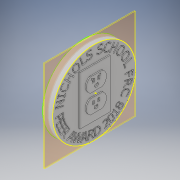
# Autodesk Inventor part: Coin Award
Saved by Autodesk Inventor 2018.2 (Build 222227000, 227)
## iProperties
Created: 2017-10-20
Part Number: Coin Award
Material: Generic
Document SubType Name: Modeling
Designer: battin.michael
Density: 1 g/cm^3
Appearance: Default
Author: battin.michael
Autodesk Inventor part; units mm, degrees
(part 1 of 3)
ref_plane "YZ Plane" through (0, 0, 0) normal (1, 0, 0) x (0, 1, 0)
ref_plane "XZ Plane" through (0, 0, 0) normal (0, 1, 0) x (-1, 0, 0)
ref_plane "XY Plane" through (0, 0, 0) normal (0, 0, 1) x (1, 0, 0)
sketch "Sketch1" plane through (0, 0, 0) normal (1, 0, 0) x (0, 1, 0)
  circle A0 centre (0, 0) radius 104.7779
  constraints: 1 centre point, 1 coincident
extrude "Extrusion1" add sketch "Sketch1" along normal blind 25.4
sketch "Sketch2" plane through (25.4, 0, 0) normal (1, 0, 0) x (0, 0, -1)
  line L0 (-38.1, 63.5) -> (38.1029, 63.5)
  line L1 (38.1029, 63.5) -> (38.1029, -60.325)
  line L2 (38.1029, -60.325) -> (-38.1, -60.325)
  line L3 (-38.1, -60.325) -> (-38.1, 63.5)
  circle A0 centre (0, 0) radius 104.7779 projected
  dimension "d56" = 66.6779
  dimension "d57" = 66.675
  constraints: 8 end point, 2 parallel, 1 horizontal, 1 perpendicular
  measures "d56" distance edge to line of A0 L3
  measures "d57" distance edge to line of A0 L1
extrude "Extrusion2" add sketch "Sketch2" along normal blind 2.54 contours L0 L1 L2 L3
sketch "Sketch3" plane through (27.94, 0, 0) normal (1, 0, 0) x (0, 0, -1)
  line L0 (-14.4399, 43.18) -> (16.0401, 43.18)
  line L1 (16.0528, 7.62) -> (-14.4272, 7.62)
  arc A0 (-14.4399, 43.18) -> (-14.4272, 7.62) centre (-4.1683, 25.4037) ccw
  arc A1 (16.0528, 7.62) -> (16.0401, 43.18) centre (5.7812, 25.3963) ccw
  line L2 (-16.0372, -4.445) -> (14.4428, -4.445) construction
  line L3 (-16.0372, -40.005) -> (14.4428, -40.005)
  arc A2 (14.4428, -40.005) -> (14.4428, -4.445) centre (4.1776, -22.225) ccw
  arc A3 (-16.0372, -4.445) -> (-16.0372, -40.005) centre (-5.7719, -22.225) ccw
  line L4 (38.1029, 63.5) -> (-38.1, 63.5) projected
  line L5 (-38.1, 63.5) -> (-38.1, -60.325) projected
  line L6 (38.1029, -60.325) -> (38.1029, 63.5) projected
  line L7 (-38.1, -60.325) -> (38.1029, -60.325) projected
  line L8 (38.1029, 63.5) -> (-38.1, 63.5) projected
  line L9 (-38.1, 63.5) -> (-38.1, -60.325) projected
  line L10 (-38.1, -60.325) -> (38.1029, -60.325) projected
  line L11 (38.1029, -60.325) -> (38.1029, 63.5) projected
  line L12 (-16.0372, -4.445) -> (14.4428, -4.445)
  line L13 (14.4428, -40.005) -> (-16.0372, -40.005)
  arc A4 (-16.0372, -4.445) -> (-16.0372, -40.005) centre (-5.7719, -22.225) ccw
  arc A5 (14.4428, -40.005) -> (14.4428, -4.445) centre (4.1776, -22.225) ccw
  point P0 (0, 0)
  dimension "d6" = 30.48
  dimension "d7" = 30.48
  dimension "d8" = 20.32
  dimension "d9" = 23.6601
  dimension "d10" = 23.6728
  dimension "d11" = 35.56
  dimension "d12" = 120
  dimension "d13" = 120
  dimension "d14" = 22.0629
  dimension "d15" = 30.48
  dimension "d16" = 30.48
  dimension "d17" = 23.6601
  dimension "d18" = 35.56
  dimension "d21" = 120
  dimension "d22" = 120
  dimension "d23" = 23.6601
  dimension "d24" = 38.1
  constraints: 12 end point, 12 point on circle, 6 centre point, 3 equal length, 3 horizontal, 1 concentric
  measures "d6" distance of L0.start L0.end
  measures "d7" distance of L1.start L1.end
  measures "d8" distance between parallel lines of L4 L0
  measures "d9" distance from line of L5 L0.start
  measures "d10" distance from line of L5 L1.end
  measures "d11" distance between parallel lines of L0 L1
  measures "d14" distance from line of L6 L0.end
  measures "d15" distance of L2.start L2.end
  measures "d16" distance of L3.start L3.end
  measures "d17" distance from line of L6 L2.end
  measures "d18" distance of L3.start L2.start
  measures "d23" distance from line of L6 L3.end
  measures "d24" distance from line of L7 A3.centre
extrude "Extrusion3" add sketch "Sketch3" along normal blind 2.54 contours L0 A1 L1 A0
ref_plane "Work Plane1" through (15.24, 0, 0) normal (1, 0, 0) x (0, 0, -1)
sketch "Sketch4" plane through (27.94, 0, 0) normal (1, 0, 0) x (0, 0, -1)
  line L0 (-14.4493, -4.4578) -> (15.0773, -4.4578)
  line L1 (16.0307, -40.005) -> (-14.4493, -40.005)
  line L2 (-38.1, -60.325) -> (38.1029, -60.325) projected
  arc A0 (16.0307, -40.005) -> (15.0773, -4.4578) centre (5.3071, -22.5062) ccw
  arc A1 (-14.4493, -4.4578) -> (-14.4493, -40.005) centre (-4.1877, -22.2314) ccw
  point P0 (0, 0)
  point P1 (16.0401, 43.18)
  dimension "d26" = 35.56
  dimension "d28" = 20.32
  dimension "d32" = 30.48
  dimension "d33" = 20.5232
  dimension "d34" = 20.5232
  dimension "d35" = 120
  dimension "d36" = 35.5472
  constraints: 4 end point, 4 point on circle, 2 centre point, 1 horizontal
  measures "d26" distance of L0.end L1.start
  measures "d28" distance between parallel lines of L2 L1
  measures "d32" distance of L1.start L1.end
  measures "d33" radius of A0
  measures "d34" radius of A1
  measures "d36" distance of L1.end L0.start
extrude "Extrusion4" [suppressed]
sketch "Sketch5" plane through (30.48, 0, 0) normal (1, 0, 0) x (0, 0, -1)
  point P0 (0, 0)
sketch "Sketch6" plane through (27.94, 0, 0) normal (1, 0, 0) x (0, 0, -1)
  line L0 (-14.4272, -4.445) -> (16.0528, -4.445)
  line L1 (16.0528, -40.005) -> (-14.4272, -40.005)
  arc A0 (-14.4272, -4.445) -> (-14.4272, -40.005) centre (-4.1767, -22.225) ccw
  arc A1 (16.0528, -40.005) -> (16.0528, -4.445) centre (5.8023, -22.225) ccw
  line L2 (38.1029, 63.5) -> (-38.1, 63.5) projected
  line L3 (38.1029, -60.325) -> (38.1029, 63.5) projected
  point P0 (0, 0)
  dimension "d37" = 35.56
  dimension "d38" = 20.5232
  dimension "d39" = 20.5232
  dimension "d42" = 103.505
  dimension "d43" = 35.56
  dimension "d44" = 30.48
  dimension "d45" = 30.48
  dimension "d58" = 22.0501
  constraints: 4 end point, 4 point on circle, 2 centre point
  measures "d37" distance of L0.end L1.start
  measures "d38" radius of A0
  measures "d39" radius of A1
  measures "d42" distance between parallel lines of L2 L1
  measures "d43" distance from line of L1 L0.start
  measures "d44" distance of L0.end L0.start
  measures "d45" distance of L1.start L1.end
  measures "d58" distance from line of L3 L0.end
extrude "Extrusion5" add sketch "Sketch6" along normal blind 2.54
sketch "Sketch7" plane through (30.48, 0, 0) normal (1, 0, 0) x (0, 0, -1)
  line L0 (-9.271, -12.3825) -> (-4.699, -12.3825)
  line L1 (-4.699, -12.3825) -> (-4.699, -20.6375)
  line L2 (-4.699, -20.6375) -> (-9.271, -20.6375)
  line L3 (-9.271, -20.6375) -> (-9.271, -12.3825)
  line L4 (-38.1, 63.5) -> (-38.1, -60.325) projected
  point P0 (0, 0)
  dimension "d46" = 4.572
  dimension "d47" = 8.255
  dimension "d50" = 28.829
  constraints: 8 end point, 2 parallel, 1 horizontal, 1 perpendicular
  measures "d46" distance of L1.end L2.end
  measures "d47" distance of L0.end L1.end
  measures "d50" distance between parallel lines of L4 L3
sketch "Sketch8" plane through (30.48, 0, 0) normal (1, 0, 0) x (0, 0, -1)
  line L0 (4.7019, -12.3237) -> (9.2739, -12.3237)
  line L1 (9.2739, -12.3237) -> (9.2739, -20.5787)
  line L2 (9.2739, -20.5787) -> (4.7019, -20.5787)
  line L3 (4.7019, -20.5787) -> (4.7019, -12.3237)
  line L4 (38.1029, -60.325) -> (38.1029, 63.5) projected
  point P0 (0, 0)
  dimension "d48" = 8.255
  dimension "d49" = 4.572
  dimension "d51" = 28.829
  constraints: 8 end point, 1 horizontal, 1 parallel, 1 perpendicular
  measures "d48" distance between parallel lines of L2 L0
  measures "d49" distance of L2.end L1.end
  measures "d51" distance between parallel lines of L4 L1
extrude "Extrusion6" cut sketch "Sketch7" against normal blind 2.54
extrude "Extrusion7" cut sketch "Sketch8" against normal blind 2.54
sketch "Sketch9" plane through (30.48, 0, 0) normal (1, 0, 0) x (0, 0, -1)
  point P0 (0, 0)
sketch "Sketch10" plane through (30.48, 0, 0) normal (1, 0, 0) x (0, 0, -1)
  line L0 (-4.7625, -25.4) -> (4.7625, -25.4)
  line L1 (4.7625, -25.4) -> (4.7625, -28.575)
  line L2 (-4.7625, -28.575) -> (-4.7625, -25.4)
  arc A0 (-4.7625, -28.575) -> (4.7625, -28.575) centre (0, -28.575) ccw
  point P0 (0, 0)
  constraints: 6 end point, 2 point on circle, 2 tangent, 1 centre point, 1 horizontal, 1 parallel, 1 perpendicular
extrude "Extrusion8" cut sketch "Sketch10" against normal blind 2.54
sketch "Sketch11" plane through (27.94, 0, 0) normal (1, 0, 0) x (0, 0, -1)
  line L0 (-1.5365, 36.5125) -> (-3.175, 36.5125)
  line L1 (-3.175, 36.5125) -> (-3.175, 28.575)
  line L2 (-3.175, 28.575) -> (-1.5365, 28.575)
  line L3 (-1.5365, 28.575) -> (-1.5365, 36.5125)
  point P0 (0, 0)
  constraints: 8 end point, 2 parallel, 1 horizontal, 1 perpendicular
sketch "Sketch12" plane through (30.48, 0, 0) normal (1, 0, 0) x (0, 0, -1)
  line L0 (-9.6418, 26.9748) -> (-4.887, 26.9748)
  line L1 (-4.887, 26.9748) -> (-4.887, 35.2298)
  line L2 (-9.6418, 35.2298) -> (-9.6418, 26.9748)
  line L3 (4.89, 26.9748) -> (9.6449, 26.9748)
  line L4 (9.6449, 26.9748) -> (9.6449, 35.2298)
  line L5 (4.89, 35.2298) -> (4.89, 26.9748)
  line L6 (16.0401, 43.18) -> (-14.4399, 43.18) projected
  line L7 (-9.6418, 35.2298) -> (-4.887, 35.2298)
  line L8 (4.89, 35.2298) -> (9.6449, 35.2298)
  point P0 (0, 0)
  dimension "d67" = 4.7549
  constraints: 16 end point, 3 equal length, 3 horizontal, 2 perpendicular, 1 point on line
  measures "d67" distance between parallel lines of L1 L2
sketch "Sketch13" plane through (30.48, 0, 0) normal (1, 0, 0) x (0, 0, -1)
  line L0 (-11.1154, 39.0904) -> (-3.164, 35.1147)
  line L1 (-3.164, 35.1147) -> (-4.8678, 31.7069)
  line L2 (-4.8678, 31.7069) -> (-12.8193, 35.6826)
  line L3 (-12.8193, 35.6826) -> (-11.1154, 39.0904)
  line L4 (-12.8193, 35.6826) -> (-9.6969, 34.1215)
  point P0 (0, 0)
  dimension "d66" = 8.89
  dimension "d68" = 3.81
  constraints: 10 end point, 2 perpendicular, 1 point on line
  measures "d66" distance between parallel lines of L1 L3
  measures "d68" distance between parallel lines of L0 L2
sketch "Sketch14" plane through (30.48, 0, 0) normal (1, 0, 0) x (0, 0, -1)
  line L0 (5.0529, 31.7537) -> (12.676, 36.3276)
  line L1 (12.676, 36.3276) -> (10.7157, 39.5946)
  line L2 (10.7157, 39.5946) -> (3.0926, 35.0208)
  line L3 (3.0926, 35.0208) -> (5.0529, 31.7537)
  point P0 (0, 0)
  dimension "d69" = 8.89
  dimension "d70" = 3.81
  constraints: 8 end point, 3 perpendicular
  measures "d69" distance between parallel lines of L1 L3
  measures "d70" distance between parallel lines of L0 L2
sketch "Sketch15" plane through (30.48, 0, 0) normal (1, 0, 0) x (0, 0, -1)
  line L0 (-4.9096, 19.5798) -> (4.568, 22.7602)
  line L1 (-4.9096, 19.5798) -> (-3.3742, 16.2781)
  line L2 (4.568, 22.7602) -> (5.7109, 19.2106)
  arc A0 (-3.3742, 16.2781) -> (5.7109, 19.2106) centre (0.987, 18.3061) ccw
  point P0 (0, 0)
  dimension "d71" = 7.091
  dimension "d72" = 3.0834
  dimension "d73" = 4.7738
  dimension "d74" = 83.612
  dimension "d75" = 89.298
  constraints: 6 end point, 2 point on circle, 1 centre point, 1 tangent
  measures "d71" angle of L2 L1
  measures "d72" distance from line of A0.centre L0
  measures "d73" distance from line of A0.centre L2
  measures "d74" angle of L0 L1
  measures "d75" angle of L2 L0
sketch "Sketch16" plane through (25.4, 0, 0) normal (1, 0, 0) x (0, 0, -1)
  point P0 (0, 0)
extrude "Extrusion9" cut sketch "Sketch15" against normal blind 2.54
extrude "Extrusion10" cut sketch "Sketch13" against normal blind 2.54
extrude "Extrusion11" cut sketch "Sketch14" against normal blind 2.54
extrude "Extrusion12" cut sketch "Sketch12" against normal blind 2.54 contours L5 L8 L4 L3
sketch "Sketch17" plane through (30.48, 0, 0) normal (1, 0, 0) x (0, 0, -1)
  line L0 (-4.7099, 31.8568) -> (-4.7099, 27.0816)
  line L1 (9.6449, 26.9748) -> (4.89, 26.9748) projected
  line L2 (-4.7099, 27.0816) -> (-9.4724, 27.0816)
  line L3 (-9.4724, 27.0816) -> (-9.4724, 34.0092)
  line L4 (-4.8678, 31.7069) -> (-12.8193, 35.6826) projected
  line L5 (-9.4724, 34.0092) -> (-4.8678, 31.7069)
  line L6 (-4.7099, 31.8568) -> (-4.7099, 32.077)
  line L7 (-4.7099, 32.077) -> (-9.4724, 34.4582)
  line L8 (-9.4724, 34.4582) -> (-9.4724, 34.0092)
  point P0 (0, 0)
  constraints: 14 end point, 3 perpendicular, 2 parallel, 1 collinear, 1 vertical
sketch "Sketch18" plane through (30.48, 0, 0) normal (1, 0, 0) x (0, 0, -1)
  point P0 (0, 0)
extrude "Extrusion13" cut sketch "Sketch17" against normal blind 2.54
ref_plane "Work Plane2" through (12.7, 0, 0) normal (1, 0, 0) x (0, 0, -1)
sketch "Sketch19" plane through (25.4, 0, 0) normal (1, 0, 0) x (0, 0, -1)
  point P0 (0, 0)
sketch "Sketch20" plane through (25.4, 0, 0) normal (1, 0, 0) x (0, 0, -1)
  circle A0 centre (0, 0) radius 88.0088
  spline S0 degree 2 poles (-64.3921, -66.344) (-64.9936, -66.9063) (-66.4769, -67.4897) (-67.2113, -67.4576) knots 0 0 0 1 2 2 2
  spline S1 degree 2 poles (-67.2113, -67.4576) (-68.1347, -67.4192) (-69.8392, -66.5753) (-70.7669, -65.5828) knots 0 0 0 1 2 2 2
  line L0 (-70.7669, -65.5828) -> (-71.7438, -64.5377)
  line L1 (-71.7438, -64.5377) -> (-75.2023, -67.7705)
  line L2 (-75.2023, -67.7705) -> (-76.3549, -66.5374)
  line L3 (-76.3549, -66.5374) -> (-67.0769, -57.8651)
  line L4 (-67.0769, -57.8651) -> (-64.8982, -60.1959)
  spline S2 degree 2 poles (-64.8982, -60.1959) (-64.1252, -61.023) (-63.3136, -62.4339) (-63.2072, -63.1656) knots 0 0 0 1 2 2 2
  spline S3 degree 2 poles (-63.2072, -63.1656) (-63.0757, -64.0147) (-63.6177, -65.6202) (-64.3921, -66.344) knots 0 0 0 1 2 2 2
  spline S4 degree 2 poles (-65.6315, -65.0935) (-65.1503, -64.6437) (-64.7528, -63.6523) (-64.8434, -63.1031) knots 0 0 0 1 2 2 2
  spline S5 degree 2 poles (-64.8434, -63.1031) (-64.922, -62.6272) (-65.495, -61.6976) (-66.0362, -61.1187) knots 0 0 0 1 2 2 2
  line L5 (-66.0362, -61.1187) -> (-66.992, -60.0962)
  line L6 (-66.992, -60.0962) -> (-70.6911, -63.5538)
  line L7 (-70.6911, -63.5538) -> (-69.904, -64.3959)
  spline S6 degree 2 poles (-69.904, -64.3959) (-69.2013, -65.1478) (-68.0962, -65.8477) (-67.4993, -65.8533) knots 0 0 0 1 2 2 2
  spline S7 degree 2 poles (-67.4993, -65.8533) (-66.9611, -65.8714) (-66.0751, -65.5081) (-65.6315, -65.0935) knots 0 0 0 1 2 2 2
  line L8 (-69.6937, -73.4893) -> (-61.2888, -63.9684)
  line L9 (-61.2888, -63.9684) -> (-55.3324, -69.2265)
  line L10 (-55.3324, -69.2265) -> (-56.3269, -70.353)
  line L11 (-56.3269, -70.353) -> (-61.0179, -66.2118)
  line L12 (-61.0179, -66.2118) -> (-63.32, -68.8197)
  line L13 (-63.32, -68.8197) -> (-58.9454, -72.6816)
  line L14 (-58.9454, -72.6816) -> (-59.9398, -73.808)
  line L15 (-59.9398, -73.808) -> (-64.3145, -69.9461)
  line L16 (-64.3145, -69.9461) -> (-67.4339, -73.4798)
  line L17 (-67.4339, -73.4798) -> (-62.7429, -77.621)
  line L18 (-62.7429, -77.621) -> (-63.7373, -78.7474)
  line L19 (-63.7373, -78.7474) -> (-69.6937, -73.4893)
  line L20 (-62.2708, -79.8763) -> (-54.8247, -69.5882)
  line L21 (-54.8247, -69.5882) -> (-48.3884, -74.2466)
  line L22 (-48.3884, -74.2466) -> (-49.2694, -75.4638)
  line L23 (-49.2694, -75.4638) -> (-54.3384, -71.795)
  line L24 (-54.3384, -71.795) -> (-56.3779, -74.613)
  line L25 (-56.3779, -74.613) -> (-51.6507, -78.0344)
  line L26 (-51.6507, -78.0344) -> (-52.5317, -79.2516)
  line L27 (-52.5317, -79.2516) -> (-57.2589, -75.8302)
  line L28 (-57.2589, -75.8302) -> (-60.0226, -79.6487)
  line L29 (-60.0226, -79.6487) -> (-54.9535, -83.3174)
  line L30 (-54.9535, -83.3174) -> (-55.8345, -84.5347)
  line L31 (-55.8345, -84.5347) -> (-62.2708, -79.8763)
  line L32 (-45.7704, -90.4564) -> (-47.6677, -89.3583)
  line L33 (-47.6677, -89.3583) -> (-48.6104, -82.9742)
  line L34 (-48.6104, -82.9742) -> (-50.285, -82.005)
  line L35 (-50.285, -82.005) -> (-52.8162, -86.3786)
  line L36 (-52.8162, -86.3786) -> (-54.277, -85.5331)
  line L37 (-54.277, -85.5331) -> (-47.9154, -74.5413)
  line L38 (-47.9154, -74.5413) -> (-45.0829, -76.1807)
  spline S8 degree 2 poles (-45.0829, -76.1807) (-44.1387, -76.7271) (-42.9835, -77.6692) (-42.621, -78.3784) knots 0 0 0 1 2 2 2
  spline S9 degree 2 poles (-42.621, -78.3784) (-42.2585, -79.0876) (-42.2658, -80.6411) (-42.7659, -81.5051) knots 0 0 0 1 2 2 2
  spline S10 degree 2 poles (-42.7659, -81.5051) (-43.4618, -82.7077) (-45.6345, -83.6263) (-46.9124, -83.4099) knots 0 0 0 1 2 2 2
  line L39 (-46.9124, -83.4099) -> (-45.7704, -90.4564)
  spline S11 degree 2 poles (-44.3561, -80.7394) (-44.0777, -80.2584) (-43.9883, -79.3232) (-44.2054, -78.8765) knots 0 0 0 1 2 2 2
  spline S12 degree 2 poles (-44.2054, -78.8765) (-44.3986, -78.4912) (-45.129, -77.8425) (-45.7347, -77.4919) knots 0 0 0 1 2 2 2
  line L40 (-45.7347, -77.4919) -> (-47.1867, -76.6516)
  line L41 (-47.1867, -76.6516) -> (-49.5787, -80.7847)
  line L42 (-49.5787, -80.7847) -> (-48.296, -81.527)
  spline S13 degree 2 poles (-48.296, -81.527) (-47.6636, -81.8931) (-46.5282, -82.2529) (-45.9797, -82.1066) knots 0 0 0 1 2 2 2
  spline S14 degree 2 poles (-45.9797, -82.1066) (-45.4838, -81.9893) (-44.686, -81.3095) (-44.3561, -80.7394) knots 0 0 0 1 2 2 2
  line L43 (-41.1552, -92.6298) -> (-32.625, -82.2927)
  line L44 (-32.625, -82.2927) -> (-30.6829, -83.0343)
  line L45 (-30.6829, -83.0343) -> (-31.2137, -96.426)
  line L46 (-31.2137, -96.426) -> (-32.8771, -95.7909)
  line L47 (-32.8771, -95.7909) -> (-32.6872, -92.0626)
  line L48 (-32.6872, -92.0626) -> (-37.2157, -90.3334)
  line L49 (-37.2157, -90.3334) -> (-39.5592, -93.2392)
  line L50 (-39.5592, -93.2392) -> (-41.1552, -92.6298)
  line L51 (-32.6059, -90.5514) -> (-32.3092, -84.2641)
  line L52 (-32.3092, -84.2641) -> (-36.2691, -89.1526)
  line L53 (-36.2691, -89.1526) -> (-32.6059, -90.5514)
  line L54 (-13.1407, -87.8693) -> (-19.1961, -99.4797)
  line L55 (-19.1961, -99.4797) -> (-21.0379, -99.0394)
  line L56 (-21.0379, -99.0394) -> (-21.1004, -88.1889)
  line L57 (-21.1004, -88.1889) -> (-25.9927, -97.8551)
  line L58 (-25.9927, -97.8551) -> (-27.8145, -97.4197)
  line L59 (-27.8145, -97.4197) -> (-28.0152, -84.3139)
  line L60 (-28.0152, -84.3139) -> (-26.3235, -84.7183)
  line L61 (-26.3235, -84.7183) -> (-26.2887, -95.5516)
  line L62 (-26.2887, -95.5516) -> (-21.3787, -85.9002)
  line L63 (-21.3787, -85.9002) -> (-19.7071, -86.2998)
  line L64 (-19.7071, -86.2998) -> (-19.7009, -97.2532)
  line L65 (-19.7009, -97.2532) -> (-14.7522, -87.4841)
  line L66 (-14.7522, -87.4841) -> (-13.1407, -87.8693)
  line L67 (-15.9288, -100.1015) -> (-10.3464, -87.9172)
  line L68 (-10.3464, -87.9172) -> (-8.2788, -88.134)
  line L69 (-8.2788, -88.134) -> (-5.3452, -101.2112)
  line L70 (-5.3452, -101.2112) -> (-7.1159, -101.0255)
  line L71 (-7.1159, -101.0255) -> (-7.892, -97.374)
  line L72 (-7.892, -97.374) -> (-12.713, -96.8685)
  line L73 (-12.713, -96.8685) -> (-14.2297, -100.2796)
  line L74 (-14.2297, -100.2796) -> (-15.9288, -100.1015)
  line L75 (-8.2024, -95.8927) -> (-9.5338, -89.7409)
  line L76 (-9.5338, -89.7409) -> (-12.1022, -95.4838)
  line L77 (-12.1022, -95.4838) -> (-8.2024, -95.8927)
  line L78 (5.8515, -101.2079) -> (3.6594, -101.2113)
  line L79 (3.6594, -101.2113) -> (-0.3621, -96.1642)
  line L80 (-0.3621, -96.1642) -> (-2.297, -96.1672)
  line L81 (-2.297, -96.1672) -> (-2.2892, -101.2204)
  line L82 (-2.2892, -101.2204) -> (-3.9771, -101.223)
  line L83 (-3.9771, -101.223) -> (-3.9965, -88.523)
  line L84 (-3.9965, -88.523) -> (-0.7238, -88.518)
  spline S15 degree 2 poles (-0.7238, -88.518) (0.3672, -88.5163) (1.8392, -88.7508) (2.5089, -89.182) knots 0 0 0 1 2 2 2
  spline S16 degree 2 poles (2.5089, -89.182) (3.1785, -89.6132) (3.9524, -90.9603) (3.954, -91.9585) knots 0 0 0 1 2 2 2
  spline S17 degree 2 poles (3.954, -91.9585) (3.9561, -93.3479) (2.5387, -95.2335) (1.325, -95.6882) knots 0 0 0 1 2 2 2
  line L85 (1.325, -95.6882) -> (5.8515, -101.2079)
  spline S18 degree 2 poles (2.1943, -92.095) (2.1934, -91.5393) (1.801, -90.6857) (1.3889, -90.4084) knots 0 0 0 1 2 2 2
  spline S19 degree 2 poles (1.3889, -90.4084) (1.0284, -90.1723) (0.0709, -89.9782) (-0.6289, -89.9793) knots 0 0 0 1 2 2 2
  line L86 (-0.6289, -89.9793) -> (-2.3065, -89.9818)
  line L87 (-2.3065, -89.9818) -> (-2.2991, -94.7572)
  line L88 (-2.2991, -94.7572) -> (-0.8171, -94.7549)
  spline S20 degree 2 poles (-0.8171, -94.7549) (-0.0864, -94.7538) (1.0761, -94.4947) (1.4769, -94.0927) knots 0 0 0 1 2 2 2
  spline S21 degree 2 poles (1.4769, -94.0927) (1.8469, -93.7422) (2.1953, -92.7537) (2.1943, -92.095) knots 0 0 0 1 2 2 2
  spline S22 degree 2 poles (16.085, -93.6581) (16.282, -95.3862) (15.198, -98.3272) (14.1106, -99.2384) knots 0 0 0 1 2 2 2
  spline S23 degree 2 poles (14.1106, -99.2384) (13.2182, -99.9512) (11.2913, -100.5851) (9.7574, -100.7599) knots 0 0 0 1 2 2 2
  line L89 (9.7574, -100.7599) -> (6.8534, -101.0909)
  line L90 (6.8534, -101.0909) -> (5.4155, -88.4725)
  line L91 (5.4155, -88.4725) -> (8.2888, -88.1451)
  spline S24 degree 2 poles (8.2888, -88.1451) (10.0681, -87.9423) (12.1533, -88.2433) (12.9227, -88.6321) knots 0 0 0 1 2 2 2
  spline S25 degree 2 poles (12.9227, -88.6321) (14.2316, -89.3013) (15.8753, -91.8175) (16.085, -93.6581) knots 0 0 0 1 2 2 2
  spline S26 degree 2 poles (14.3341, -93.8369) (14.1687, -92.3849) (12.9733, -90.4391) (11.9559, -89.9646) knots 0 0 0 1 2 2 2
  spline S27 degree 2 poles (11.9559, -89.9646) (11.2355, -89.6427) (9.6711, -89.4584) (8.5361, -89.5878) knots 0 0 0 1 2 2 2
  line L92 (8.5361, -89.5878) -> (7.2579, -89.7334)
  line L93 (7.2579, -89.7334) -> (8.3649, -99.4477)
  line L94 (8.3649, -99.4477) -> (9.6431, -99.3021)
  spline S28 degree 2 poles (9.6431, -99.3021) (10.7577, -99.1751) (12.4041, -98.6249) (13.0345, -98.0662) knots 0 0 0 1 2 2 2
  spline S29 degree 2 poles (13.0345, -98.0662) (13.8463, -97.3729) (14.5019, -95.3094) (14.3341, -93.8369) knots 0 0 0 1 2 2 2
  line L95 (31.1198, -96.3968) -> (23.5775, -98.5072)
  line L96 (23.5775, -98.5072) -> (23.0921, -96.7728)
  spline S30 degree 2 poles (23.0921, -96.7728) (23.6913, -95.7822) (24.7417, -93.9601) (25.222, -93.0028) knots 0 0 0 1 2 2 2
  spline S31 degree 2 poles (25.222, -93.0028) (26.1896, -91.0755) (26.6946, -88.9464) (26.42, -87.9652) knots 0 0 0 1 2 2 2
  spline S32 degree 2 poles (26.42, -87.9652) (26.2758, -87.4499) (25.7424, -86.7656) (25.3856, -86.5982) knots 0 0 0 1 2 2 2
  spline S33 degree 2 poles (25.3856, -86.5982) (25.0289, -86.4309) (24.2063, -86.3938) (23.7504, -86.5214) knots 0 0 0 1 2 2 2
  spline S34 degree 2 poles (23.7504, -86.5214) (23.3143, -86.6434) (22.4833, -87.1111) (22.1241, -87.3933) knots 0 0 0 1 2 2 2
  spline S35 degree 2 poles (22.1241, -87.3933) (21.816, -87.6291) (21.2828, -88.2058) (21.1234, -88.4) knots 0 0 0 1 2 2 2
  line L97 (21.1234, -88.4) -> (21.0342, -88.425)
  line L98 (21.0342, -88.425) -> (20.5461, -86.6806)
  spline S36 degree 2 poles (20.5461, -86.6806) (20.9822, -86.2914) (22.66, -85.2983) (23.4727, -85.0709) knots 0 0 0 1 2 2 2
  spline S37 degree 2 poles (23.4727, -85.0709) (25.1873, -84.5911) (27.6275, -85.864) (28.0601, -87.4101) knots 0 0 0 1 2 2 2
  spline S38 degree 2 poles (28.0601, -87.4101) (28.2626, -88.1336) (28.2639, -89.4371) (28.1108, -90.0357) knots 0 0 0 1 2 2 2
  spline S39 degree 2 poles (28.1108, -90.0357) (27.9632, -90.6541) (27.3949, -91.9459) (27.0607, -92.5845) knots 0 0 0 1 2 2 2
  spline S40 degree 2 poles (27.0607, -92.5845) (26.5233, -93.6432) (25.135, -95.9767) (24.7171, -96.6601) knots 0 0 0 1 2 2 2
  line L99 (24.7171, -96.6601) -> (30.7232, -94.9795)
  line L100 (30.7232, -94.9795) -> (31.1198, -96.3968)
  spline S41 degree 2 poles (37.8276, -87.0936) (39.0534, -90.2831) (38.3475, -93.9833) (36.4166, -94.7254) knots 0 0 0 1 2 2 2
  spline S42 degree 2 poles (36.4166, -94.7254) (34.4568, -95.4786) (31.4516, -93.1385) (30.2516, -90.0163) knots 0 0 0 1 2 2 2
  spline S43 degree 2 poles (30.2516, -90.0163) (29.0185, -86.8077) (29.7317, -83.1267) (31.6722, -82.3809) knots 0 0 0 1 2 2 2
  spline S44 degree 2 poles (31.6722, -82.3809) (33.6224, -81.6314) (36.6387, -84.0003) (37.8276, -87.0936) knots 0 0 0 1 2 2 2
  spline S45 degree 2 poles (37.1792, -91.4885) (37.1845, -90.8139) (36.6826, -88.934) (36.2137, -87.7139) knots 0 0 0 1 2 2 2
  spline S46 degree 2 poles (36.2137, -87.7139) (35.7448, -86.4939) (34.8622, -84.7713) (34.3894, -84.2583) knots 0 0 0 1 2 2 2
  spline S47 degree 2 poles (34.3894, -84.2583) (33.9167, -83.7454) (32.8409, -83.4422) (32.178, -83.697) knots 0 0 0 1 2 2 2
  spline S48 degree 2 poles (32.178, -83.697) (31.5152, -83.9517) (30.9002, -84.9048) (30.8904, -85.6252) knots 0 0 0 1 2 2 2
  spline S49 degree 2 poles (30.8904, -85.6252) (30.8828, -86.3227) (31.4188, -88.2336) (31.8655, -89.396) knots 0 0 0 1 2 2 2
  spline S50 degree 2 poles (31.8655, -89.396) (32.3455, -90.6449) (33.1416, -92.2574) (33.6425, -92.8147) knots 0 0 0 1 2 2 2
  spline S51 degree 2 poles (33.6425, -92.8147) (34.1093, -93.3409) (35.2191, -93.6751) (35.9108, -93.4093) knots 0 0 0 1 2 2 2
  spline S52 degree 2 poles (35.9108, -93.4093) (36.564, -93.1582) (37.179, -92.2052) (37.1792, -91.4885) knots 0 0 0 1 2 2 2
  line L101 (48.0313, -89.1576) -> (42.4825, -91.9138)
  line L102 (42.4825, -91.9138) -> (41.9056, -90.7524)
  line L103 (41.9056, -90.7524) -> (43.9703, -89.7268)
  line L104 (43.9703, -89.7268) -> (40.1841, -82.1041)
  line L105 (40.1841, -82.1041) -> (38.1194, -83.1297)
  line L106 (38.1194, -83.1297) -> (37.602, -82.0881)
  spline S53 degree 2 poles (37.602, -82.0881) (38.7726, -81.5067) (39.5491, -80.2936) (39.165, -79.3352) knots 0 0 0 1 2 2 2
  line L107 (39.165, -79.3352) -> (40.3448, -78.7492)
  line L108 (40.3448, -78.7492) -> (45.4359, -88.9989)
  line L109 (45.4359, -88.9989) -> (47.4545, -87.9962)
  line L110 (47.4545, -87.9962) -> (48.0313, -89.1576)
  spline S54 degree 2 poles (53.4956, -86.264) (52.6909, -86.763) (51.0719, -87.101) (50.3317, -86.9424) knots 0 0 0 1 2 2 2
  spline S55 degree 2 poles (50.3317, -86.9424) (49.6057, -86.7871) (48.3957, -85.8905) (47.9781, -85.217) knots 0 0 0 1 2 2 2
  spline S56 degree 2 poles (47.9781, -85.217) (47.4357, -84.3424) (47.4603, -82.2926) (48.0812, -81.302) knots 0 0 0 1 2 2 2
  line L111 (48.0812, -81.302) -> (48.0541, -81.2583)
  spline S57 degree 2 poles (48.0541, -81.2583) (46.9707, -81.2883) (45.5176, -80.6636) (45.0077, -79.8414) knots 0 0 0 1 2 2 2
  spline S58 degree 2 poles (45.0077, -79.8414) (44.2538, -78.6256) (45.0817, -75.8598) (46.4986, -74.9811) knots 0 0 0 1 2 2 2
  spline S59 degree 2 poles (46.4986, -74.9811) (47.968, -74.0699) (50.6982, -74.5082) (51.4467, -75.7152) knots 0 0 0 1 2 2 2
  spline S60 degree 2 poles (51.4467, -75.7152) (51.8969, -76.4411) (51.9272, -78.3842) (51.3807, -79.2801) knots 0 0 0 1 2 2 2
  line L112 (51.3807, -79.2801) -> (51.4079, -79.3238)
  spline S61 degree 2 poles (51.4079, -79.3238) (52.6237, -79.1753) (54.3756, -79.8328) (54.9939, -80.8299) knots 0 0 0 1 2 2 2
  spline S62 degree 2 poles (54.9939, -80.8299) (55.8509, -82.2118) (55, -85.3311) (53.4956, -86.264) knots 0 0 0 1 2 2 2
  spline S63 degree 2 poles (53.5938, -81.8919) (53.1816, -81.2272) (52.1686, -80.7654) (51.1757, -80.8241) knots 0 0 0 1 2 2 2
  spline S64 degree 2 poles (51.1757, -80.8241) (50.844, -80.8361) (49.8212, -81.0223) (49.1749, -81.1324) knots 0 0 0 1 2 2 2
  spline S65 degree 2 poles (49.1749, -81.1324) (48.8243, -81.8948) (48.9126, -83.4628) (49.3736, -84.2062) knots 0 0 0 1 2 2 2
  spline S66 degree 2 poles (49.3736, -84.2062) (49.9811, -85.1858) (51.9538, -85.7306) (52.8459, -85.1773) knots 0 0 0 1 2 2 2
  spline S67 degree 2 poles (52.8459, -85.1773) (53.7555, -84.6132) (54.1796, -82.8365) (53.5938, -81.8919) knots 0 0 0 1 2 2 2
  spline S68 degree 2 poles (50.0406, -76.6113) (49.5904, -75.8854) (48.0175, -75.5166) (47.1516, -76.0536) knots 0 0 0 1 2 2 2
  spline S69 degree 2 poles (47.1516, -76.0536) (46.3644, -76.5417) (45.8956, -78.0314) (46.3566, -78.7748) knots 0 0 0 1 2 2 2
  spline S70 degree 2 poles (46.3566, -78.7748) (46.6875, -79.3084) (47.6645, -79.7318) (48.365, -79.7092) knots 0 0 0 1 2 2 2
  spline S71 degree 2 poles (48.365, -79.7092) (48.6596, -79.696) (49.8525, -79.5496) (50.3045, -79.4389) knots 0 0 0 1 2 2 2
  spline S72 degree 2 poles (50.3045, -79.4389) (50.6359, -78.5673) (50.4474, -77.2673) (50.0406, -76.6113) knots 0 0 0 1 2 2 2
  line L113 (-52.1152, 71.0647) -> (-53.5825, 69.8676)
  line L114 (-53.5825, 69.8676) -> (-64.859, 74.8001)
  line L115 (-64.859, 74.8001) -> (-57.9365, 66.3153)
  line L116 (-57.9365, 66.3153) -> (-59.1566, 65.3199)
  line L117 (-59.1566, 65.3199) -> (-67.1851, 75.1603)
  line L118 (-67.1851, 75.1603) -> (-65.327, 76.6762)
  line L119 (-65.327, 76.6762) -> (-55.0073, 72.1187)
  line L120 (-55.0073, 72.1187) -> (-61.3638, 79.9097)
  line L121 (-61.3638, 79.9097) -> (-60.1437, 80.9051)
  line L122 (-60.1437, 80.9051) -> (-52.1152, 71.0647)
  line L123 (-46.2675, 74.9059) -> (-50.3792, 72.205)
  line L124 (-50.3792, 72.205) -> (-51.0911, 73.2888)
  line L125 (-51.0911, 73.2888) -> (-49.7406, 74.1759)
  line L126 (-49.7406, 74.1759) -> (-55.2893, 82.623)
  line L127 (-55.2893, 82.623) -> (-56.6398, 81.7359)
  line L128 (-56.6398, 81.7359) -> (-57.3518, 82.8197)
  line L129 (-57.3518, 82.8197) -> (-53.2401, 85.5206)
  line L130 (-53.2401, 85.5206) -> (-52.5281, 84.4368)
  line L131 (-52.5281, 84.4368) -> (-53.8786, 83.5496)
  line L132 (-53.8786, 83.5496) -> (-48.3299, 75.1026)
  line L133 (-48.3299, 75.1026) -> (-46.9794, 75.9897)
  line L134 (-46.9794, 75.9897) -> (-46.2675, 74.9059)
  spline S73 degree 2 poles (-40.0131, 78.139) (-41.1059, 77.5635) (-43.3429, 77.3277) (-44.4051, 77.7105) knots 0 0 0 1 2 2 2
  spline S74 degree 2 poles (-44.4051, 77.7105) (-45.4626, 78.0841) (-47.3511, 79.8812) (-48.0992, 81.3018) knots 0 0 0 1 2 2 2
  spline S75 degree 2 poles (-48.0992, 81.3018) (-48.8425, 82.7133) (-49.226, 85.1866) (-48.9506, 86.3202) knots 0 0 0 1 2 2 2
  spline S76 degree 2 poles (-48.9506, 86.3202) (-48.6747, 87.4309) (-47.2525, 89.1918) (-46.1142, 89.7912) knots 0 0 0 1 2 2 2
  spline S77 degree 2 poles (-46.1142, 89.7912) (-45.5496, 90.0885) (-44.4707, 90.4473) (-43.9846, 90.5404) knots 0 0 0 1 2 2 2
  spline S78 degree 2 poles (-43.9846, 90.5404) (-43.5581, 90.6138) (-42.6248, 90.6749) (-42.146, 90.6712) knots 0 0 0 1 2 2 2
  line L135 (-42.146, 90.6712) -> (-41.1965, 88.8681)
  line L136 (-41.1965, 88.8681) -> (-41.3149, 88.8058)
  spline S79 degree 2 poles (-41.3149, 88.8058) (-41.6111, 88.8824) (-42.4989, 89.0663) (-43.0746, 89.0772) knots 0 0 0 1 2 2 2
  spline S80 degree 2 poles (-43.0746, 89.0772) (-43.6272, 89.0886) (-44.7963, 88.8568) (-45.4519, 88.5115) knots 0 0 0 1 2 2 2
  spline S81 degree 2 poles (-45.4519, 88.5115) (-46.1713, 88.1327) (-47.1436, 86.8647) (-47.329, 86.0459) knots 0 0 0 1 2 2 2
  spline S82 degree 2 poles (-47.329, 86.0459) (-47.5004, 85.2229) (-47.1126, 83.2054) (-46.542, 82.1218) knots 0 0 0 1 2 2 2
  spline S83 degree 2 poles (-46.542, 82.1218) (-45.933, 80.9653) (-44.5, 79.5914) (-43.7152, 79.2718) knots 0 0 0 1 2 2 2
  spline S84 degree 2 poles (-43.7152, 79.2718) (-42.9492, 78.9657) (-41.3861, 79.0676) (-40.6758, 79.4417) knots 0 0 0 1 2 2 2
  spline S85 degree 2 poles (-40.6758, 79.4417) (-40.0293, 79.7821) (-39.0952, 80.6811) (-38.7919, 81.1432) knots 0 0 0 1 2 2 2
  spline S86 degree 2 poles (-38.7919, 81.1432) (-38.5068, 81.5958) (-38.1556, 82.4088) (-38.0737, 82.6729) knots 0 0 0 1 2 2 2
  line L137 (-38.0737, 82.6729) -> (-37.9645, 82.7305)
  line L138 (-37.9645, 82.7305) -> (-37.0246, 80.9456)
  spline S87 degree 2 poles (-37.0246, 80.9456) (-37.3068, 80.576) (-37.7946, 79.912) (-38.1823, 79.5218) knots 0 0 0 1 2 2 2
  spline S88 degree 2 poles (-38.1823, 79.5218) (-38.5878, 79.0989) (-39.3392, 78.4938) (-40.0131, 78.139) knots 0 0 0 1 2 2 2
  line L139 (-26.5432, 84.0373) -> (-28.1239, 83.4454)
  line L140 (-28.1239, 83.4454) -> (-30.3036, 89.2669)
  line L141 (-30.3036, 89.2669) -> (-35.7781, 87.217)
  line L142 (-35.7781, 87.217) -> (-33.5984, 81.3955)
  line L143 (-33.5984, 81.3955) -> (-35.179, 80.8037)
  line L144 (-35.179, 80.8037) -> (-39.6324, 92.6973)
  line L145 (-39.6324, 92.6973) -> (-38.0518, 93.2891)
  line L146 (-38.0518, 93.2891) -> (-36.305, 88.6242)
  line L147 (-36.305, 88.6242) -> (-30.8305, 90.6741)
  line L148 (-30.8305, 90.6741) -> (-32.5772, 95.339)
  line L149 (-32.5772, 95.339) -> (-30.9966, 95.9308)
  line L150 (-30.9966, 95.9308) -> (-26.5432, 84.0373)
  spline S89 degree 2 poles (-17.7919, 97.7357) (-16.9038, 97.0704) (-15.5786, 94.8368) (-15.2307, 93.2905) knots 0 0 0 1 2 2 2
  spline S90 degree 2 poles (-15.2307, 93.2905) (-14.892, 91.7844) (-15.1062, 89.1728) (-15.6439, 88.1868) knots 0 0 0 1 2 2 2
  spline S91 degree 2 poles (-15.6439, 88.1868) (-16.2128, 87.1517) (-18.0458, 85.8743) (-19.2607, 85.601) knots 0 0 0 1 2 2 2
  spline S92 degree 2 poles (-19.2607, 85.601) (-20.5158, 85.3187) (-22.716, 85.7205) (-23.6364, 86.389) knots 0 0 0 1 2 2 2
  spline S93 degree 2 poles (-23.6364, 86.389) (-24.5346, 87.052) (-25.842, 89.3001) (-26.1853, 90.8263) knots 0 0 0 1 2 2 2
  spline S94 degree 2 poles (-26.1853, 90.8263) (-26.5354, 92.3827) (-26.2953, 94.9262) (-25.7744, 95.9401) knots 0 0 0 1 2 2 2
  spline S95 degree 2 poles (-25.7744, 95.9401) (-25.2366, 96.926) (-23.4104, 98.2335) (-22.1653, 98.5136) knots 0 0 0 1 2 2 2
  spline S96 degree 2 poles (-22.1653, 98.5136) (-20.9002, 98.7981) (-18.6732, 98.3708) (-17.7919, 97.7357) knots 0 0 0 1 2 2 2
  spline S97 degree 2 poles (-16.9477, 92.9043) (-17.2233, 94.1293) (-18.1823, 95.9073) (-18.8043, 96.4214) knots 0 0 0 1 2 2 2
  spline S98 degree 2 poles (-18.8043, 96.4214) (-19.4409, 96.9533) (-20.9711, 97.2843) (-21.8346, 97.09) knots 0 0 0 1 2 2 2
  spline S99 degree 2 poles (-21.8346, 97.09) (-22.7282, 96.889) (-23.9336, 95.9638) (-24.2967, 95.1859) knots 0 0 0 1 2 2 2
  spline S100 degree 2 poles (-24.2967, 95.1859) (-24.6464, 94.4427) (-24.7394, 92.4175) (-24.4683, 91.2126) knots 0 0 0 1 2 2 2
  spline S101 degree 2 poles (-24.4683, 91.2126) (-23.9195, 88.7727) (-21.2884, 86.6429) (-19.5714, 87.0291) knots 0 0 0 1 2 2 2
  spline S102 degree 2 poles (-19.5714, 87.0291) (-17.8544, 87.4153) (-16.3989, 90.4644) (-16.9477, 92.9043) knots 0 0 0 1 2 2 2
  line L151 (-4.6682, 87.9901) -> (-11.9886, 87.242)
  line L152 (-11.9886, 87.242) -> (-13.2798, 99.8761)
  line L153 (-13.2798, 99.8761) -> (-11.6007, 100.0478)
  line L154 (-11.6007, 100.0478) -> (-10.4623, 88.9084)
  line L155 (-10.4623, 88.9084) -> (-4.8209, 89.4849)
  line L156 (-4.8209, 89.4849) -> (-4.6682, 87.9901)
  spline S103 degree 2 poles (0.1976, 87.7821) (-1.1815, 87.7858) (-3.1148, 88.3673) (-3.9679, 88.7812) knots 0 0 0 1 2 2 2
  line L157 (-3.9679, 88.7812) -> (-3.9623, 90.9013)
  line L158 (-3.9623, 90.9013) -> (-3.8388, 90.901)
  spline S104 degree 2 poles (-3.8388, 90.901) (-3.0072, 90.1166) (-0.8997, 89.2465) (0.078, 89.2439) knots 0 0 0 1 2 2 2
  spline S105 degree 2 poles (0.078, 89.2439) (1.4776, 89.2402) (2.9113, 90.3993) (2.9138, 91.3564) knots 0 0 0 1 2 2 2
  spline S106 degree 2 poles (2.9138, 91.3564) (2.9158, 92.118) (2.1671, 93.0669) (1.3547, 93.3057) knots 0 0 0 1 2 2 2
  spline S107 degree 2 poles (1.3547, 93.3057) (0.7685, 93.472) (-0.2086, 93.701) (-0.9389, 93.8882) knots 0 0 0 1 2 2 2
  spline S108 degree 2 poles (-0.9389, 93.8882) (-1.5971, 94.0649) (-2.6351, 94.5925) (-3.0354, 95.0156) knots 0 0 0 1 2 2 2
  spline S109 degree 2 poles (-3.0354, 95.0156) (-3.4253, 95.4386) (-3.8546, 96.5718) (-3.8526, 97.3128) knots 0 0 0 1 2 2 2
  spline S110 degree 2 poles (-3.8526, 97.3128) (-3.8485, 98.8566) (-1.4347, 100.9394) (0.4281, 100.9344) knots 0 0 0 1 2 2 2
  spline S111 degree 2 poles (0.4281, 100.9344) (1.4985, 100.9316) (3.391, 100.5046) (4.203, 100.101) knots 0 0 0 1 2 2 2
  line L159 (4.203, 100.101) -> (4.1976, 98.0838)
  line L160 (4.1976, 98.0838) -> (4.0741, 98.0842)
  spline S112 degree 2 poles (4.0741, 98.0842) (3.4684, 98.6415) (1.5769, 99.4699) (0.5374, 99.4727) knots 0 0 0 1 2 2 2
  spline S113 degree 2 poles (0.5374, 99.4727) (-0.6358, 99.4758) (-2.0899, 98.3785) (-2.0923, 97.4831) knots 0 0 0 1 2 2 2
  spline S114 degree 2 poles (-2.0923, 97.4831) (-2.0944, 96.6803) (-1.2427, 95.7209) (-0.4406, 95.5027) knots 0 0 0 1 2 2 2
  spline S115 degree 2 poles (-0.4406, 95.5027) (0.0942, 95.3572) (1.6473, 94.9825) (2.1615, 94.8268) knots 0 0 0 1 2 2 2
  spline S116 degree 2 poles (2.1615, 94.8268) (3.4674, 94.4219) (4.6776, 92.8029) (4.6744, 91.6193) knots 0 0 0 1 2 2 2
  spline S117 degree 2 poles (4.6744, 91.6193) (4.6724, 90.868) (4.0614, 89.4288) (3.5146, 88.926) knots 0 0 0 1 2 2 2
  spline S118 degree 2 poles (3.5146, 88.926) (2.9059, 88.3718) (1.3605, 87.779) (0.1976, 87.7821) knots 0 0 0 1 2 2 2
  spline S119 degree 2 poles (15.2495, 86.4476) (13.8914, 86.6878) (12.0865, 87.5922) (11.317, 88.1463) knots 0 0 0 1 2 2 2
  line L161 (11.317, 88.1463) -> (11.6862, 90.234)
  line L162 (11.6862, 90.234) -> (11.8078, 90.2125)
  spline S120 degree 2 poles (11.8078, 90.2125) (12.4925, 89.2972) (14.4195, 88.0785) (15.3823, 87.9083) knots 0 0 0 1 2 2 2
  spline S121 degree 2 poles (15.3823, 87.9083) (16.7606, 87.6645) (18.3718, 88.5606) (18.5385, 89.5032) knots 0 0 0 1 2 2 2
  spline S122 degree 2 poles (18.5385, 89.5032) (18.6711, 90.2531) (18.0961, 91.3163) (17.3367, 91.691) knots 0 0 0 1 2 2 2
  spline S123 degree 2 poles (17.3367, 91.691) (16.7877, 91.9553) (15.8644, 92.3485) (15.1771, 92.6581) knots 0 0 0 1 2 2 2
  spline S124 degree 2 poles (15.1771, 92.6581) (14.5589, 92.9451) (13.6267, 93.643) (13.305, 94.1284) knots 0 0 0 1 2 2 2
  spline S125 degree 2 poles (13.305, 94.1284) (12.9933, 94.612) (12.7648, 95.802) (12.8938, 96.5317) knots 0 0 0 1 2 2 2
  spline S126 degree 2 poles (12.8938, 96.5317) (13.1626, 98.0519) (15.8979, 99.6899) (17.7322, 99.3655) knots 0 0 0 1 2 2 2
  spline S127 degree 2 poles (17.7322, 99.3655) (18.7862, 99.1791) (20.5775, 98.4339) (21.3082, 97.8971) knots 0 0 0 1 2 2 2
  line L163 (21.3082, 97.8971) -> (20.957, 95.9107)
  line L164 (20.957, 95.9107) -> (20.8354, 95.9322)
  spline S128 degree 2 poles (20.8354, 95.9322) (20.3342, 96.5852) (18.6128, 97.7257) (17.5893, 97.9067) knots 0 0 0 1 2 2 2
  spline S129 degree 2 poles (17.5893, 97.9067) (16.4339, 98.111) (14.8132, 97.2793) (14.6573, 96.3976) knots 0 0 0 1 2 2 2
  spline S130 degree 2 poles (14.6573, 96.3976) (14.5175, 95.6071) (15.192, 94.5158) (15.9449, 94.1632) knots 0 0 0 1 2 2 2
  spline S131 degree 2 poles (15.9449, 94.1632) (16.4468, 93.9282) (17.9126, 93.2927) (18.3924, 93.0511) knots 0 0 0 1 2 2 2
  spline S132 degree 2 poles (18.3924, 93.0511) (19.6096, 92.4283) (20.5242, 90.6257) (20.3181, 89.4602) knots 0 0 0 1 2 2 2
  spline S133 degree 2 poles (20.3181, 89.4602) (20.1873, 88.7204) (19.3384, 87.4073) (18.7135, 87.0057) knots 0 0 0 1 2 2 2
  spline S134 degree 2 poles (18.7135, 87.0057) (18.0188, 86.5641) (16.3947, 86.2451) (15.2495, 86.4476) knots 0 0 0 1 2 2 2
  spline S135 degree 2 poles (26.0399, 83.8372) (24.8564, 84.19) (23.0924, 85.5857) (22.6007, 86.6022) knots 0 0 0 1 2 2 2
  spline S136 degree 2 poles (22.6007, 86.6022) (22.1061, 87.6088) (22.0129, 90.214) (22.4715, 91.7526) knots 0 0 0 1 2 2 2
  spline S137 degree 2 poles (22.4715, 91.7526) (22.9273, 93.2814) (24.3827, 95.3175) (25.3723, 95.9354) knots 0 0 0 1 2 2 2
  spline S138 degree 2 poles (25.3723, 95.9354) (26.3462, 96.5364) (28.5943, 96.8005) (29.8271, 96.433) knots 0 0 0 1 2 2 2
  spline S139 degree 2 poles (29.8271, 96.433) (30.4386, 96.2507) (31.4607, 95.7527) (31.8733, 95.4794) knots 0 0 0 1 2 2 2
  spline S140 degree 2 poles (31.8733, 95.4794) (32.2296, 95.2335) (32.9394, 94.6246) (33.2791, 94.287) knots 0 0 0 1 2 2 2
  line L165 (33.2791, 94.287) -> (32.6969, 92.3342)
  line L166 (32.6969, 92.3342) -> (32.5687, 92.3724)
  spline S141 degree 2 poles (32.5687, 92.3724) (32.4105, 92.6344) (31.9045, 93.3866) (31.5006, 93.797) knots 0 0 0 1 2 2 2
  spline S142 degree 2 poles (31.5006, 93.797) (31.1135, 94.1916) (30.1158, 94.8435) (29.4056, 95.0551) knots 0 0 0 1 2 2 2
  spline S143 degree 2 poles (29.4056, 95.0551) (28.6265, 95.2874) (27.0447, 95.0609) (26.3397, 94.6053) knots 0 0 0 1 2 2 2
  spline S144 degree 2 poles (26.3397, 94.6053) (25.6416, 94.1368) (24.508, 92.4235) (24.1581, 91.2498) knots 0 0 0 1 2 2 2
  spline S145 degree 2 poles (24.1581, 91.2498) (23.7847, 89.9973) (23.8482, 88.013) (24.1857, 87.2358) knots 0 0 0 1 2 2 2
  spline S146 degree 2 poles (24.1857, 87.2358) (24.5192, 86.4813) (25.7079, 85.4611) (26.4772, 85.2318) knots 0 0 0 1 2 2 2
  spline S147 degree 2 poles (26.4772, 85.2318) (27.1774, 85.023) (28.4737, 85.0125) (29.0137, 85.1307) knots 0 0 0 1 2 2 2
  spline S148 degree 2 poles (29.0137, 85.1307) (29.534, 85.2548) (30.3536, 85.5904) (30.5969, 85.722) knots 0 0 0 1 2 2 2
  line L167 (30.5969, 85.722) -> (30.7152, 85.6867)
  line L168 (30.7152, 85.6867) -> (30.1389, 83.7536)
  spline S149 degree 2 poles (30.1389, 83.7536) (29.6787, 83.6867) (28.8657, 83.5532) (28.3156, 83.5454) knots 0 0 0 1 2 2 2
  spline S150 degree 2 poles (28.3156, 83.5454) (27.7301, 83.5266) (26.7698, 83.6196) (26.0399, 83.8372) knots 0 0 0 1 2 2 2
  line L169 (39.7933, 78.6339) -> (38.2495, 79.3162)
  line L170 (38.2495, 79.3162) -> (40.7623, 85.0019)
  line L171 (40.7623, 85.0019) -> (35.4155, 87.3649)
  line L172 (35.4155, 87.3649) -> (32.9027, 81.6792)
  line L173 (32.9027, 81.6792) -> (31.3589, 82.3615)
  line L174 (31.3589, 82.3615) -> (36.4927, 93.9777)
  line L175 (36.4927, 93.9777) -> (38.0365, 93.2954)
  line L176 (38.0365, 93.2954) -> (36.0229, 88.7393)
  line L177 (36.0229, 88.7393) -> (41.3697, 86.3763)
  line L178 (41.3697, 86.3763) -> (43.3833, 90.9323)
  line L179 (43.3833, 90.9323) -> (44.9271, 90.2501)
  line L180 (44.9271, 90.2501) -> (39.7933, 78.6339)
  spline S151 degree 2 poles (55.6283, 82.3062) (55.7979, 81.2096) (55.1832, 78.6862) (54.3506, 77.3377) knots 0 0 0 1 2 2 2
  spline S152 degree 2 poles (54.3506, 77.3377) (53.5395, 76.0241) (51.5601, 74.3071) (50.4862, 73.9783) knots 0 0 0 1 2 2 2
  spline S153 degree 2 poles (50.4862, 73.9783) (49.3557, 73.6362) (47.1522, 74.0049) (46.0926, 74.6592) knots 0 0 0 1 2 2 2
  spline S154 degree 2 poles (46.0926, 74.6592) (44.9979, 75.335) (43.7062, 77.1608) (43.5157, 78.2823) knots 0 0 0 1 2 2 2
  spline S155 degree 2 poles (43.5157, 78.2823) (43.3373, 79.3843) (43.9749, 81.9056) (44.7967, 83.2367) knots 0 0 0 1 2 2 2
  spline S156 degree 2 poles (44.7967, 83.2367) (45.6348, 84.594) (47.5852, 86.2443) (48.6665, 86.6048) knots 0 0 0 1 2 2 2
  spline S157 degree 2 poles (48.6665, 86.6048) (49.7404, 86.9335) (51.9601, 86.5911) (53.046, 85.9206) knots 0 0 0 1 2 2 2
  spline S158 degree 2 poles (53.046, 85.9206) (54.1494, 85.2393) (55.4424, 83.3765) (55.6283, 82.3062) knots 0 0 0 1 2 2 2
  spline S159 degree 2 poles (52.8531, 78.2622) (53.5128, 79.3306) (54.0706, 81.2722) (53.9855, 82.0747) knots 0 0 0 1 2 2 2
  spline S160 degree 2 poles (53.9855, 82.0747) (53.9024, 82.9001) (53.04, 84.2067) (52.2869, 84.6717) knots 0 0 0 1 2 2 2
  spline S161 degree 2 poles (52.2869, 84.6717) (51.5076, 85.1529) (49.9989, 85.3345) (49.1954, 85.0323) knots 0 0 0 1 2 2 2
  spline S162 degree 2 poles (49.1954, 85.0323) (48.4257, 84.7456) (46.943, 83.3629) (46.2942, 82.3121) knots 0 0 0 1 2 2 2
  spline S163 degree 2 poles (46.2942, 82.3121) (44.9803, 80.1842) (45.3717, 76.8218) (46.8691, 75.8972) knots 0 0 0 1 2 2 2
  spline S164 degree 2 poles (46.8691, 75.8972) (48.3666, 74.9726) (51.5392, 76.1343) (52.8531, 78.2622) knots 0 0 0 1 2 2 2
  spline S165 degree 2 poles (66.5851, 73.7241) (66.5998, 72.6146) (65.6385, 70.2018) (64.6255, 68.9829) knots 0 0 0 1 2 2 2
  spline S166 degree 2 poles (64.6255, 68.9829) (63.6389, 67.7956) (61.4389, 66.372) (60.3296, 66.1966) knots 0 0 0 1 2 2 2
  spline S167 degree 2 poles (60.3296, 66.1966) (59.1624, 66.0158) (57.032, 66.6889) (56.0742, 67.4848) knots 0 0 0 1 2 2 2
  spline S168 degree 2 poles (56.0742, 67.4848) (55.0848, 68.307) (54.0609, 70.2953) (54.029, 71.4325) knots 0 0 0 1 2 2 2
  spline S169 degree 2 poles (54.029, 71.4325) (54.0064, 72.5486) (54.9901, 74.9561) (55.9899, 76.1592) knots 0 0 0 1 2 2 2
  spline S170 degree 2 poles (55.9899, 76.1592) (57.0095, 77.3861) (59.1713, 78.7476) (60.2924, 78.9534) knots 0 0 0 1 2 2 2
  spline S171 degree 2 poles (60.2924, 78.9534) (61.4017, 79.1289) (63.5518, 78.4795) (64.5333, 77.6639) knots 0 0 0 1 2 2 2
  spline S172 degree 2 poles (64.5333, 77.6639) (65.5306, 76.8351) (66.5507, 74.8098) (66.5851, 73.7241) knots 0 0 0 1 2 2 2
  spline S173 degree 2 poles (63.272, 70.1077) (64.0745, 71.0733) (64.8982, 72.918) (64.9261, 73.7244) knots 0 0 0 1 2 2 2
  spline S174 degree 2 poles (64.9261, 73.7244) (64.9592, 74.5533) (64.2879, 75.9677) (63.6071, 76.5333) knots 0 0 0 1 2 2 2
  spline S175 degree 2 poles (63.6071, 76.5333) (62.9027, 77.1188) (61.4342, 77.5094) (60.5964, 77.3225) knots 0 0 0 1 2 2 2
  spline S176 degree 2 poles (60.5964, 77.3225) (59.7941, 77.1461) (58.1328, 75.9843) (57.3434, 75.0344) knots 0 0 0 1 2 2 2
  spline S177 degree 2 poles (57.3434, 75.0344) (55.745, 73.111) (55.6627, 69.727) (57.0162, 68.6022) knots 0 0 0 1 2 2 2
  spline S178 degree 2 poles (57.0162, 68.6022) (58.3697, 67.4774) (61.6736, 68.1842) (63.272, 70.1077) knots 0 0 0 1 2 2 2
  line L181 (66.8699, 57.38) -> (61.811, 62.7239)
  line L182 (61.811, 62.7239) -> (71.0338, 71.4549)
  line L183 (71.0338, 71.4549) -> (72.1942, 70.2291)
  line L184 (72.1942, 70.2291) -> (64.0626, 62.5312)
  line L185 (64.0626, 62.5312) -> (67.9611, 58.413)
  line L186 (67.9611, 58.413) -> (66.8699, 57.38)
  line L187 (84.5808, 52.0257) -> (81.2694, 56.9178)
  line L188 (81.2694, 56.9178) -> (78.3035, 54.9102)
  line L189 (78.3035, 54.9102) -> (81.4764, 50.2227)
  line L190 (81.4764, 50.2227) -> (80.2321, 49.3804)
  line L191 (80.2321, 49.3804) -> (77.0592, 54.068)
  line L192 (77.0592, 54.068) -> (71.9966, 50.6412)
  line L193 (71.9966, 50.6412) -> (71.0505, 52.0389)
  line L194 (71.0505, 52.0389) -> (81.5677, 59.1578)
  line L195 (81.5677, 59.1578) -> (85.8252, 52.868)
  line L196 (85.8252, 52.868) -> (84.5808, 52.0257)
  line L197 (77.4439, 41.8177) -> (87.3478, 47.042)
  line L198 (87.3478, 47.042) -> (85.3599, 50.8106)
  line L199 (85.3599, 50.8106) -> (86.6889, 51.5117)
  line L200 (86.6889, 51.5117) -> (91.4523, 42.4816)
  line L201 (91.4523, 42.4816) -> (90.1233, 41.7806)
  line L202 (90.1233, 41.7806) -> (88.1353, 45.5492)
  line L203 (88.1353, 45.5492) -> (78.2314, 40.3248)
  line L204 (78.2314, 40.3248) -> (77.4439, 41.8177)
  spline S179 degree 2 poles (82.2674, 30.6401) (81.8232, 31.7925) (81.8495, 34.0417) (82.3534, 35.0522) knots 0 0 0 1 2 2 2
  spline S180 degree 2 poles (82.3534, 35.0522) (82.8476, 36.059) (84.8525, 37.7253) (86.3505, 38.3028) knots 0 0 0 1 2 2 2
  spline S181 degree 2 poles (86.3505, 38.3028) (87.8389, 38.8766) (90.3401, 38.9695) (91.434, 38.5639) knots 0 0 0 1 2 2 2
  spline S182 degree 2 poles (91.434, 38.5639) (92.5049, 38.1606) (94.0882, 36.5429) (94.551, 35.3425) knots 0 0 0 1 2 2 2
  spline S183 degree 2 poles (94.551, 35.3425) (94.7805, 34.7472) (95.0112, 33.6338) (95.047, 33.1403) knots 0 0 0 1 2 2 2
  spline S184 degree 2 poles (95.047, 33.1403) (95.0703, 32.708) (95.0222, 31.774) (94.9628, 31.2989) knots 0 0 0 1 2 2 2
  line L205 (94.9628, 31.2989) -> (93.0614, 30.5658)
  line L206 (93.0614, 30.5658) -> (93.0133, 30.6907)
  spline S185 degree 2 poles (93.0133, 30.6907) (93.1239, 30.976) (93.4099, 31.8363) (93.4878, 32.4068) knots 0 0 0 1 2 2 2
  spline S186 degree 2 poles (93.4878, 32.4068) (93.5635, 32.9544) (93.4694, 34.1425) (93.2029, 34.8339) knots 0 0 0 1 2 2 2
  spline S187 degree 2 poles (93.2029, 34.8339) (92.9104, 35.5925) (91.7642, 36.7059) (90.9726, 36.9853) knots 0 0 0 1 2 2 2
  spline S188 degree 2 poles (90.9726, 36.9853) (90.1752, 37.2514) (88.1263, 37.1013) (86.9836, 36.6607) knots 0 0 0 1 2 2 2
  spline S189 degree 2 poles (86.9836, 36.6607) (85.764, 36.1906) (84.2325, 34.9273) (83.8237, 34.1851) knots 0 0 0 1 2 2 2
  spline S190 degree 2 poles (83.8237, 34.1851) (83.4305, 33.46) (83.3497, 31.8956) (83.6384, 31.1466) knots 0 0 0 1 2 2 2
  spline S191 degree 2 poles (83.6384, 31.1466) (83.9013, 30.4648) (84.6853, 29.4324) (85.109, 29.0774) knots 0 0 0 1 2 2 2
  spline S192 degree 2 poles (85.109, 29.0774) (85.5253, 28.7415) (86.2919, 28.298) (86.5447, 28.1859) knots 0 0 0 1 2 2 2
  line L207 (86.5447, 28.1859) -> (86.5891, 28.0707)
  line L208 (86.5891, 28.0707) -> (84.7069, 27.345)
  spline S193 degree 2 poles (84.7069, 27.345) (84.3727, 27.6684) (83.77, 28.2303) (83.4276, 28.6608) knots 0 0 0 1 2 2 2
  spline S194 degree 2 poles (83.4276, 28.6608) (83.0548, 29.1127) (82.5414, 29.9295) (82.2674, 30.6401) knots 0 0 0 1 2 2 2
  constraints: 1 centre point, 1 coincident, 2 other